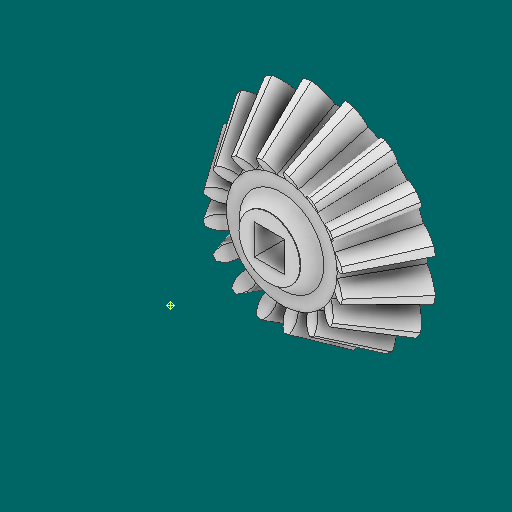
# Autodesk Inventor part: Bevel Gear1
Saved by Autodesk Inventor 2023.1 (Build 271208000, 208)
## iProperties
CustomPartVersion: 1
Created: 2022-10-29
Part Number: Bevel Gear1
Material: ABS Plastic
Document SubType Name: Modeling
Designer: zac-h
Categories: <?xml version="1.0" encoding="UTF-16"?> <MemberInstance><Categories><FamilyTemplate><FamilyTemplateParameter ValueType="xs:double" Id="1" ObjectReferenceKey="da_z" ObjectType="kUserParameterObject"/><FamilyTemplateParameter ValueType="xs:double" Id="2" ObjectReferenceKey="da_b" ObjectType="kUserParameterObject"/><FamilyTemplateParameter ValueType="xs:double" Id="3" ObjectReferenceKey="da_beta" ObjectType="kUserParameterObject"/><FamilyTemplateParameter ValueType="xs:double" Id="4" ObjectReferenceKey="da_dae" ObjectType="kUserParameterObject"/><FamilyTemplateParameter ValueType="xs:double" Id="5" ObjectReferenceKey="da_ve" ObjectType="kUserParameterObject"/><FamilyTemplateParameter ValueType="xs:double" Id="6" ObjectReferenceKey="da_omega" ObjectType="kUserParameterObject"/><FamilyTemplateParameter ValueType="xs:string" Id="7" ObjectReferenceKey="EAIAABAAAAAAHwAAAAAAAIAAAAAAAAAA" ObjectType="83914240" SubObjectId="SurfaceGeometry"/></FamilyTemplate><ParamToTemplateMap><ParamToTemplate CategoryParameter="//CategoryParameter[@InternalName='046C89C9-8512-4d59-83FE-43B91F4F132A']" TemplateParameter="1"/><ParamToTemplate CategoryParameter="//CategoryParameter[@InternalName='2552DF32-E462-4b46-AEBF-C6C7768E72AC']" TemplateParameter="2"/><ParamToTemplate CategoryParameter="//CategoryParameter[@InternalName='C9EE641D-15FC-4fae-A226-E94C4372FDD7']" TemplateParameter="3"/><ParamToTemplate><ParamToTemplate CategoryParameter="//CategoryParameter[@InternalName='00B6519A-459B-49c7-AD84-2E56D39A5744']" ConstantValue="0.000000"/></ParamToTemplate><ParamToTemplate><ParamToTemplate CategoryParameter="//CategoryParameter[@InternalName='04B31F0E-C7A6-4894-AA32-9629BEFACF47']" ConstantValue="1.000000"/></ParamToTemplate><ParamToTemplate><ParamToTemplate CategoryParameter="//CategoryParameter[@InternalName='43CBEC2E-7847-49e7-A936-2F7889FCB2D9']" ConstantValue="0.200000"/></ParamToTemplate><ParamToTemplate><ParamToTemplate CategoryParameter="//CategoryParameter[@InternalName='B1EFC894-105D-4ebd-86BF-FA20ED196853']" ConstantValue="0.266800"/></ParamToTemplate><ParamToTemplate><ParamToTemplate CategoryParameter="//CategoryParameter[@InternalName='51175063-3D10-4879-93E8-6246FE8B403D']" ConstantValue="2061532430.657340"/></ParamToTemplate><ParamToTemplate><ParamToTemplate CategoryParameter="//CategoryParameter[@InternalName='A3A52E27-4454-46a9-B0BD-C932399B70AF']" ConstantValue="0.300000"/></ParamToTemplate><ParamToTemplate CategoryParameter="//CategoryParameter[@InternalName='2A200944-5A8C-41ca-B96E-8520D2E510F1']" TemplateParameter="4"/><ParamToTemplate><ParamToTemplate CategoryParameter="//CategoryParameter[@InternalName='1A637F62-92C8-44bc-B81F-10802510B579']" ConstantValue="1.461733"/></ParamToTemplate><ParamToTemplate CategoryParameter="//CategoryParameter[@InternalName='B52DD4BE-6863-48fb-BF58-89EF6F9EC65C']" TemplateParameter="5"/><ParamToTemplate><ParamToTemplate CategoryParameter="//CategoryParameter[@InternalName='3956BFF2-84D2-457d-93C2-9B0613DEBA67']" ConstantValue="1.071534"/></ParamToTemplate><ParamToTemplate CategoryParameter="//CategoryParameter[@InternalName='739CFA02-461B-4bf8-8049-181FCAD8B28F']" TemplateParameter="6"/><ParamToTemplate><ParamToTemplate CategoryParameter="//CategoryParameter[@InternalName='A27E999F-E2CE-4481-8A2A-EBF499C4C3C5']" ConstantValue="0.000000"/></ParamToTemplate><ParamToTemplate><ParamToTemplate CategoryParameter="//CategoryParameter[@InternalName='9E1B4470-B2D3-4ff1-B813-535BB4CDF51A']" ConstantValue="3523220.976809"/></ParamToTemplate><ParamToTemplate><ParamToTemplate CategoryParameter="//CategoryParameter[@InternalName='F8452263-BFF6-458c-9FB1-07C4B99E95CD']" ConstantValue="11397033.805607"/></ParamToTemplate><ParamToTemplate><ParamToTemplate CategoryParameter="//CategoryParameter[@InternalName='3E3BB259-FD49-497f-8171-6EBC954A3479']" ConstantValue="2.000000"/></ParamToTemplate><ParamToTemplate CategoryParameter="//CategoryParameter[@InternalName='27C3BAF2-7550-4e4b-AE2C-0DB134B7D9B7']" TemplateParameter="7"/></ParamToTemplateMap><Category DisplayName="Gear" InternalName="DC85795E-93AB-48d5-8EEE-5A27447B64BD" Mnemonic="Gear"><CategoryParameter DisplayName="z" InternalName="046C89C9-8512-4d59-83FE-43B91F4F132A" Mnemonic="z"/><CategoryParameter DisplayName="b" InternalName="2552DF32-E462-4b46-AEBF-C6C7768E72AC" Mnemonic="b"/><CategoryParameter DisplayName="||b|" InternalName="C9EE641D-15FC-4fae-A226-E94C4372FDD7" Mnemonic="beta"/><CategoryParameter DisplayName="x" InternalName="00B6519A-459B-49c7-AD84-2E56D39A5744" Mnemonic="x"/><CategoryParameter DisplayName="a*" InternalName="04B31F0E-C7A6-4894-AA32-9629BEFACF47" Mnemonic="a"/><CategoryParameter DisplayName="c*" InternalName="43CBEC2E-7847-49e7-A936-2F7889FCB2D9" Mnemonic="c"/><CategoryParameter DisplayName="r|.f|*" InternalName="B1EFC894-105D-4ebd-86BF-FA20ED196853" Mnemonic="rf"/><CategoryParameter DisplayName="E" InternalName="51175063-3D10-4879-93E8-6246FE8B403D" Mnemonic="E"/><CategoryParameter DisplayName="||m|" InternalName="A3A52E27-4454-46a9-B0BD-C932399B70AF" Mnemonic="mi"/><Category DisplayName="BevelGear" InternalName="0C98F69A-0C2B-4791-B2FE-7691BB227E77" Mnemonic="BevelGear"><CategoryParameter DisplayName="d|.ae|" InternalName="2A200944-5A8C-41ca-B96E-8520D2E510F1" Mnemonic="dae"/><CategoryParameter DisplayName="d|.ai|" InternalName="1A637F62-92C8-44bc-B81F-10802510B579" Mnemonic="dai"/><CategoryParameter DisplayName="A|.e|" InternalName="B52DD4BE-6863-48fb-BF58-89EF6F9EC65C" Mnemonic="ve"/><CategoryParameter DisplayName="A|.i|" InternalName="3956BFF2-84D2-457d-93C2-9B0613DEBA67" Mnemonic="vi"/><CategoryParameter DisplayName="||S|" InternalName="739CFA02-461B-4bf8-8049-181FCAD8B28F" Mnemonic="omega"/><CategoryParameter DisplayName="x|.t|" InternalName="A27E999F-E2CE-4481-8A2A-EBF499C4C3C5" Mnemonic="xt"/><CategoryParameter DisplayName="||s||.Flim|" InternalName="9E1B4470-B2D3-4ff1-B813-535BB4CDF51A" Mnemonic="sFlim"/><CategoryParameter DisplayName="||s||.Hlim|" InternalName="F8452263-BFF6-458c-9FB1-07C4B99E95CD" Mnemonic="sHlim"/><CategoryParameter DisplayName="type" InternalName="3E3BB259-FD49-497f-8171-6EBC954A3479" Mnemonic="type"/><CategoryParameter DisplayName="PitchDiameter" InternalName="27C3BAF2-7550-4e4b-AE2C-0DB134B7D9B7" Mnemonic="IDS_PITCHDIAM"/></Category></Category></Categories></MemberInstance>
Mass: 60.9118 g
Surface Area: 34.3074 cm^2
Volume: 7.7496 cm^3
Density: 1.06 g/cm^3
Appearance: Smooth - White
d48: 0.0000 in
d49: 0.0000 in
d50: 90.00 deg
d52: 0.0000 in
d53: 0.0000 in
d54: 0.00 deg
Author: zac-h
Autodesk Inventor part; units mm, degrees
ref_plane "Mesh Plane2" through (0, 0, 0) normal (0.9807853, 0.1950903, 0) x (0, 0, 1)
sketch "Teeth Body Sketch" plane through (0, 0, 0) normal (1, 0, 0) x (0, 1, 0)
  line L0 (0, 0) -> (8.848916, -17.921939) construction
  line L1 (8.848916, -17.921939) -> (11.25257, -16.497551)
  line L2 (11.25257, -16.497551) -> (0, 0) construction
  line L3 (10.16, -17.145) -> (0, 0) construction
  line L4 (5.747467, -11.640494) -> (7.308667, -10.715338)
  line L5 (8.848916, -17.921939) -> (5.747467, -11.640494)
  line L6 (11.25257, -16.497551) -> (7.308667, -10.715338)
  line L7 (0, -19.302436) -> (0, 3.217073)
  line L8 (0, -17.145) -> (11.25257, -17.145) construction
  dimension "d0" = 20.32
  dimension "d1" = 17.69783
  dimension "d2" = 22.50514
  dimension "d3" = 6.985
  dimension "d4" = 16.49755
  constraints: 16 end point, 4 point on line, 3 perpendicular, 2 collinear, 1 horizontal alignment, 1 vertical alignment
  measures "d0" diameter of L3.start L7
  measures "d1" diameter of L0.end L7
  measures "d2" diameter of L1.end L7
  measures "d3" distance between parallel lines of L1 L4
  measures "d4" vertical distance of L1.end L0.start
revolve "Teeth Body" add sketch "Teeth Body Sketch" angle 360 about axis through (0, 0, 0) along (0, 0, 1)
ref_plane "Tooth Plane" through (0, 10.16, -17.145) normal (0, -0.5098024, 0.8602915) x (1, 0, 0)
sketch "Start Sketch" plane through (0, 10.16, -17.145) normal (0, -0.5098024, 0.8602915) x (1, 0, 0)
  line L0 (0, -15.083706) -> (0, 5.026636)
  arc A0 (-0.800527, -1.85928) -> (-2.719863, 1.839857) centre (-4.274671, -1.314373) ccw
  arc A1 (2.719863, 1.839857) -> (0.800527, -1.85928) centre (4.274671, -1.314373) ccw
  line L1 (-0.800527, -1.85928) -> (0.800527, -1.85928)
  arc A2 (2.719863, 1.839857) -> (-2.719863, 1.839857) centre (0, -11.80995) ccw
  dimension "d7" = 3.51662
  dimension "d8" = 4.27467
  dimension "d9" = 10.49558
  dimension "d57" = 13.91815
  dimension "d58" = 9.95067
  constraints: 6 point on circle, 3 centre point, 3 symmetric about line, 2 end point, 1 coincident, 1 perpendicular, 1 other
  measures "d7" radius of A0
  measures "d8" horizontal distance of point (0, -11.81) A0.centre
  measures "d9" vertical distance of point (0, -11.81) A0.centre
  measures "d57" radius of A2
  measures "d58" distance from line of A2.centre L1
sketch "End Sketch" plane through (0, 6.527811, -11.015681) normal (0, -0.5098024, 0.8602915) x (1, 0, 0)
  line L0 (0, -9.216393) -> (0, 3.071358)
  arc A0 (-0.51434, -1.194589) -> (-1.747515, 1.18211) centre (-2.746481, -0.844486) ccw
  arc A1 (1.747515, 1.18211) -> (0.51434, -1.194589) centre (2.746481, -0.844486) ccw
  line L1 (-0.51434, -1.194589) -> (0.51434, -1.194589)
  arc A2 (1.747515, 1.18211) -> (-1.747515, 1.18211) centre (0, -7.587906) ccw
  dimension "d12" = 2.25943
  dimension "d15" = 2.74648
  dimension "d16" = 6.74342
  dimension "d59" = 8.94243
  dimension "d60" = 6.39332
  constraints: 6 point on circle, 3 centre point, 3 symmetric about line, 2 end point, 1 coincident, 1 other
  measures "d12" radius of A0
  measures "d15" horizontal distance of A0.centre point (0, -7.588)
  measures "d16" vertical distance of A0.centre point (0, -7.588)
  measures "d59" radius of A2
  measures "d60" distance from line of A2.centre L1
loft "Loft" cut profiles "Start Sketch", "End Sketch"
pattern_circular "Circular Pattern" count 16 over 360 about axis through (0, 0, 0) along (0, 0, 1) of "Loft"
ref_plane "End Plane" through (0, 6.527811, -11.015681) normal (0, -0.5098024, 0.8602915) x (1, 0, 0)
sketch3d "3D Sketch Right"
ref_plane "End Plane Right" through (-1.716953, 6.297967, -11.015681) normal (0.1340889, -0.4918523, 0.8602915) x (0.96479, 0.2630213, 0)
sketch "End Sketch Right" plane through (-1.716953, 6.297967, -11.015681) normal (0.1340889, -0.4918523, 0.8602915) x (0.96479, 0.2630213, 0)
  arc A0 (-0.51434, -1.194589) -> (-1.747515, 1.18211) centre (-2.746481, -0.844486) ccw
  line L0 (0, -11.002691) -> (0, 4.730751)
  arc A1 (1.747515, 1.18211) -> (0.51434, -1.194589) centre (2.746481, -0.844486) ccw
  line L1 (-0.51434, -1.194589) -> (0.51434, -1.194589)
  arc A2 (1.747515, 1.18211) -> (-1.747515, 1.18211) centre (0, -7.587906) ccw
  dimension "d70" = 2.74648
  dimension "d71" = 6.74342
  dimension "d72" = 2.25943
  dimension "d73" = 6.39332
  dimension "d74" = 8.94243
  constraints: 6 point on circle, 3 centre point, 3 symmetric about line, 2 end point, 1 coincident, 1 perpendicular, 1 other
  measures "d70" horizontal distance of A2.centre A0.centre
  measures "d71" vertical distance of point (0, -7.588) A0.centre
  measures "d72" radius of A0
  measures "d73" distance from line of point (0, -7.588) L1
  measures "d74" radius of A2
feature "Loft Right" [suppressed]
pattern_circular "Circular Pattern Right" [suppressed]
sketch3d "3D Sketch Left"
ref_plane "End Plane Left" through (1.583259, 6.297967, -10.979793) normal (-0.1241144, -0.4937085, 0.860725) x (0.969824, -0.2438061, 0)
sketch "End Sketch Left" plane through (1.583259, 6.297967, -10.979793) normal (-0.1241144, -0.4937085, 0.860725) x (0.969824, -0.2438061, 0)
  line L0 (0, -17.13005) -> (0, 7.694814)
  arc A0 (-0.51434, -1.183692) -> (-1.747515, 1.193008) centre (-2.746481, -0.833589) ccw
  arc A1 (1.747515, 1.193008) -> (0.51434, -1.183692) centre (2.746481, -0.833589) ccw
  line L1 (-0.51434, -1.183692) -> (0.51434, -1.183692)
  ellipse E0 centre (0, -5.45486) end of major axis (7.308667, -5.45486) minor radius 6.290752
  arc A2 (1.747515, 1.193008) -> (-1.747515, 1.193008) centre (0, -7.577008) ccw
  dimension "d56" = 6.29075
  dimension "d30" = 2.25943
  dimension "d31" = 2.74648
  dimension "d32" = 6.74342
  dimension "d61" = 8.94243
  dimension "d62" = 6.39332
  constraints: 6 point on circle, 3 centre point, 3 symmetric about line, 2 end point, 1 coincident, 2 other
  measures "d30" radius of A0
  measures "d31" horizontal distance of point (0, -7.577) A0.centre
  measures "d32" vertical distance of A0.centre point (0, -7.577)
  measures "d61" radius of A2
  measures "d62" distance from line of point (0, -7.577) L1
feature "Loft Left" [suppressed]
pattern_circular "Circular Pattern Left" [suppressed]
sketch "Body Sketch" plane through (0, 0, 0) normal (1, 0, 0) x (0, 1, 0)
  line L0 (0, -17.312214) -> (0, -8.724256)
  line L1 (8.848916, -17.921939) -> (5.747467, -11.640494)
  line L2 (5.747467, -11.640494) -> (0, -11.640494)
  line L3 (8.848916, -17.921939) -> (0, -17.921939)
  constraints: 4 end point, 2 perpendicular, 2 point on line
sketch "Body Sketch outline for Fix Body" plane through (0, 0, 0) normal (1, 0, 0) x (0, 1, 0)
  line L0 (0, -17.921939) -> (8.848916, -17.921939)
  line L1 (0, -11.640494) -> (0, -17.921939)
  line L2 (5.747467, -11.640494) -> (0, -11.640494)
  line L3 (8.848916, -17.921939) -> (5.747467, -11.640494)
revolve "Fix Body" add sketch "Body Sketch outline for Fix Body" angle 360 about axis through (0, 0, 0) along (0, 0, 1)
sketch "Sketch6" plane through (0, 0, 0) normal (1, 0, 0) x (0, 1, 0)
  line L0 (10.16, -17.145) -> (0, 0) projected
  line L1 (0, -18.288) -> (0, 3.048) projected
surface revolve "Pitch Diameter" sketch "Sketch6" angle 360 about axis through (0, 0, 0) along (0, 0, 1) shown no curves L0
sketch "Sketch8" plane through (0, 0, -11.640494) normal (0, 0, 1) x (1, 0, 0)
  circle A0 centre (0, 0) radius 3.175
  line L0 (1.5875, 1.5875) -> (-1.5875, 1.5875)
  line L1 (-1.5875, 1.5875) -> (-1.5875, -1.5875)
  line L2 (-1.5875, -1.5875) -> (1.5875, -1.5875)
  line L3 (1.5875, -1.5875) -> (1.5875, 1.5875)
  line L4 (1.5875, 1.5875) -> (-1.5875, -1.5875) construction
  line L5 (-1.5875, 1.5875) -> (1.5875, -1.5875) construction
  dimension "d90" = 6.35
  dimension "d91" = 3.175
  dimension "d92" = 3.175
  constraints: 12 end point, 2 midpoint, 2 parallel, 1 centre point, 1 coincident, 1 horizontal, 1 perpendicular
  measures "d90" diameter of A0
  measures "d91" distance of L2.end L1.end
  measures "d92" distance of L1.end L0.end
ref_plane "Work Plane6" through (-12.7, -5.796955, -7.9375) normal (0, 0, -1) x (0, 1, 0)
ref_plane "Work Plane7" through (-12.7, -5.796955, -7.62) normal (0, 0, -1) x (0, 1, 0)
extrude "Extrusion1" add sketch "Sketch8" along normal blind 1.27
extrude "Extrusion2" cut sketch "Sketch8" along normal through all both and the other way through all contours L3 L2 L1 L0
chamfer "Chamfer1" distance 1.2 angle 45 1 edges at (-3.175, 0, -11.6405)
equation "\"d0\" = da_de"
equation "\"d1\" = da_dfe"
equation "\"d2\" = da_dae"
equation "\"d3\" = da_b"
equation "\"d4\" = da_ve"
equation "\"d7\" = fd_rr"
equation "\"d8\" = fd_x"
equation "\"d9\" = fd_y"
equation "\"d57\" = 0.5 * fd_dva + 0.3 * da_he"
equation "\"d58\" = 0.5 * fd_dva - 1.12 * da_he"
equation "\"da_teethtype\" = 0"
equation "\"da_b\" = 6.985"
equation "\"da_de\" = 20.32"
equation "\"da_dae\" = 22.50514"
equation "\"da_dfe\" = 17.69783"
equation "\"da_le\" = 19.92929"
equation "\"da_omega\" = 90deg"
equation "\"da_beta\" = 0"
equation "\"da_delta\" = 30.650668deg"
equation "\"da_alpha\" = 14.5deg"
equation "\"da_he\" = 2.794"
equation "\"da_ve\" = 16.49755"
equation "\"da_zv\" = 18.598346"
equation "\"fd_loft\" = da_b + 0.05 * da_he"
equation "\"fd_x\" = fd_x1 + fd_x2"
equation "\"fd_y\" = fd_y1 - fd_y2"
equation "\"fd_dd\" = fd_dva - 0.8 * da_he"
equation "\"da_dvw\" = 23.6199"
equation "\"d11\" = fd_loft"
equation "\"da_dm\" = 16.75903"
equation "\"da_x\" = 0"
equation "\"da_m\" = 1.27"
equation "\"d50\" = da_omega"
equation "\"fd_rr\" = 3.516618"
equation "\"fd_dva\" = 26.1599"
equation "\"fd_x1\" = 0.99627"
equation "\"fd_x2\" = 3.278401"
equation "\"fd_y1\" = 11.767853"
equation "\"fd_y2\" = 1.272276"
body "Solid1"
body "Srf1"
